Autodesk Fusion 360 part; units mm, degrees
(part 6 of 10)
sketch "草图16 (8)" plane through (0, 0, 19.8) normal (0, 0, 1) x (1, 0, 0) in component "R1_Integrated"
  line L0 (589, 140) -> (725, 140)
  line L1 (725, 140) -> (725, 167)
  line L2 (725, 167) -> (589, 167)
  line L3 (589, 167) -> (589, 140)
  dimension "d2412" = 589
  dimension "d2414" = 136
  dimension "d2415" = 27
  constraint horizontal L0
  constraint vertical L1
  constraint horizontal L2
  constraint vertical L3
  measures "d2412" horizontal distance of origin L0.start
  measures "d2414" horizontal distance of L0.start L0.end
  measures "d2415" vertical distance of L0.end L1.end
extrude "R02 remove projecting spout''" cut sketch "草图16 (8)" along normal blind 20.4 bodies 13 in component "R1_Integrated"
ref_plane "工作平面17" through (593, 0, 0) normal (1, 0, 0) x (0, 1, 0) in component "R1_Integrated"
sketch "草图17 (8)" plane through (593, 0, 0) normal (1, 0, 0) x (0, 0, -1) in component "R1_Integrated"
  line L0 (-24.9649, 136.9) -> (-24.6782, 141)
  line L1 (-24.6782, 141) -> (-41, 141)
  line L2 (-41, 141) -> (-41, 136.9)
  line L3 (-41, 136.9) -> (-24.9649, 136.9)
  dimension "d2420" = 24.9649
  dimension "d2421" = 136.9
  dimension "d2422" = 24.6782
  dimension "d2423" = 141
  dimension "d2424" = 41
  constraint horizontal L1
  constraint vertical L2
  constraint horizontal L3
  measures "d2420" horizontal distance of origin L0.start
  measures "d2421" vertical distance of origin L0.start
  measures "d2422" horizontal distance of origin L0.end
  measures "d2423" vertical distance of origin L0.end
  measures "d2424" horizontal distance of origin L1.end
extrude "R02 full width open front''" cut sketch "草图17 (8)" along normal blind 128 bodies 13 in component "R1_Integrated"
ref_plane "工作平面14" through (0, 0, 36) normal (0, 0, 1) x (1, 0, 0) in component "R1_RemovableGrate"
sketch "草图14 (13)" plane through (0, 0, 36) normal (0, 0, 1) x (1, 0, 0) in component "R1_RemovableGrate"
  line L0 (592.7, 59.7) -> (595.3, 59.7)
  line L1 (595.3, 59.7) -> (595.3, 65.3)
  line L2 (595.3, 65.3) -> (592.7, 65.3)
  line L3 (592.7, 65.3) -> (592.7, 59.7)
  dimension "d2430" = 59.7
  dimension "d2431" = 2.6
  dimension "d2432" = 5.6
  constraint horizontal L0
  constraint vertical L1
  constraint horizontal L2
  constraint vertical L3
  measures "d2430" vertical distance of origin L0.start
  measures "d2431" horizontal distance of L0.start L0.end
  measures "d2432" vertical distance of L0.end L1.end
extrude "R02 side locating notch 0''" cut sketch "草图14 (13)" along normal blind 4 bodies 14 in component "R1_RemovableGrate"
ref_plane "工作平面18" through (0, 0, 20) normal (0, 0, 1) x (1, 0, 0) in component "R1_Integrated"
sketch "草图18 (4)" plane through (0, 0, 20) normal (0, 0, 1) x (1, 0, 0) in component "R1_Integrated"
  line L0 (593, 60) -> (595, 60)
  line L1 (595, 60) -> (595, 65)
  line L2 (595, 65) -> (593, 65)
  line L3 (593, 65) -> (593, 60)
  dimension "d2438" = 60
  dimension "d2439" = 2
  dimension "d2440" = 5
  constraint horizontal L0
  constraint vertical L1
  constraint horizontal L2
  constraint vertical L3
  measures "d2438" vertical distance of origin L0.start
  measures "d2439" horizontal distance of L0.start L0.end
  measures "d2440" vertical distance of L0.end L1.end
extrude "R02 side locating key 0''" add sketch "草图18 (4)" along normal blind 20 bodies 13 in component "R1_Integrated"
ref_plane "工作平面15" through (0, 0, 36) normal (0, 0, 1) x (1, 0, 0) in component "R1_RemovableGrate"
sketch "草图15 (13)" plane through (0, 0, 36) normal (0, 0, 1) x (1, 0, 0) in component "R1_RemovableGrate"
  line L0 (718.7, 59.7) -> (721.3, 59.7)
  line L1 (721.3, 59.7) -> (721.3, 65.3)
  line L2 (721.3, 65.3) -> (718.7, 65.3)
  line L3 (718.7, 65.3) -> (718.7, 59.7)
  dimension "d2445" = 718.7
  dimension "d2446" = 59.7
  dimension "d2447" = 2.6
  dimension "d2448" = 5.6
  constraint horizontal L0
  constraint vertical L1
  constraint horizontal L2
  constraint vertical L3
  measures "d2445" horizontal distance of origin L0.start
  measures "d2446" vertical distance of origin L0.start
  measures "d2447" horizontal distance of L0.start L0.end
  measures "d2448" vertical distance of L0.end L1.end
extrude "R02 side locating notch 1''" cut sketch "草图15 (13)" along normal blind 4 bodies 14 in component "R1_RemovableGrate"
ref_plane "工作平面19" through (0, 0, 20) normal (0, 0, 1) x (1, 0, 0) in component "R1_Integrated"
sketch "草图19 (4)" plane through (0, 0, 20) normal (0, 0, 1) x (1, 0, 0) in component "R1_Integrated"
  line L0 (719, 60) -> (721, 60)
  line L1 (721, 60) -> (721, 65)
  line L2 (721, 65) -> (719, 65)
  line L3 (719, 65) -> (719, 60)
  dimension "d2453" = 719
  dimension "d2454" = 60
  dimension "d2455" = 2
  dimension "d2456" = 5
  constraint horizontal L0
  constraint vertical L1
  constraint horizontal L2
  constraint vertical L3
  measures "d2453" horizontal distance of origin L0.start
  measures "d2454" vertical distance of origin L0.start
  measures "d2455" horizontal distance of L0.start L0.end
  measures "d2456" vertical distance of L0.end L1.end
extrude "R02 side locating key 1''" add sketch "草图19 (4)" along normal blind 20 bodies 13 in component "R1_Integrated"
ref_plane "工作平面16" through (0, 0, 19.8) normal (0, 0, 1) x (1, 0, 0) in component "R2_Integrated"
sketch "草图16 (9)" plane through (0, 0, 19.8) normal (0, 0, 1) x (1, 0, 0) in component "R2_Integrated"
  line L0 (725, 140) -> (861, 140)
  line L1 (861, 140) -> (861, 167)
  line L2 (861, 167) -> (725, 167)
  line L3 (725, 167) -> (725, 140)
  dimension "d2461" = 725
  dimension "d2463" = 136
  dimension "d2464" = 27
  constraint horizontal L0
  constraint vertical L1
  constraint horizontal L2
  constraint vertical L3
  measures "d2461" horizontal distance of origin L0.start
  measures "d2463" horizontal distance of L0.start L0.end
  measures "d2464" vertical distance of L0.end L1.end
extrude "R02 remove projecting spout'''" cut sketch "草图16 (9)" along normal blind 20.4 bodies 19 in component "R2_Integrated"
ref_plane "工作平面17" through (729, 0, 0) normal (1, 0, 0) x (0, 1, 0) in component "R2_Integrated"
sketch "草图17 (9)" plane through (729, 0, 0) normal (1, 0, 0) x (0, 0, -1) in component "R2_Integrated"
  line L0 (-24.9649, 136.9) -> (-24.6782, 141)
  line L1 (-24.6782, 141) -> (-41, 141)
  line L2 (-41, 141) -> (-41, 136.9)
  line L3 (-41, 136.9) -> (-24.9649, 136.9)
  dimension "d2469" = 24.9649
  dimension "d2470" = 136.9
  dimension "d2471" = 24.6782
  dimension "d2472" = 141
  dimension "d2473" = 41
  constraint horizontal L1
  constraint vertical L2
  constraint horizontal L3
  measures "d2469" horizontal distance of origin L0.start
  measures "d2470" vertical distance of origin L0.start
  measures "d2471" horizontal distance of origin L0.end
  measures "d2472" vertical distance of origin L0.end
  measures "d2473" horizontal distance of origin L1.end
extrude "R02 full width open front'''" cut sketch "草图17 (9)" along normal blind 128 bodies 19 in component "R2_Integrated"
ref_plane "工作平面14" through (0, 0, 36) normal (0, 0, 1) x (1, 0, 0) in component "R2_RemovableGrate"
sketch "草图14 (14)" plane through (0, 0, 36) normal (0, 0, 1) x (1, 0, 0) in component "R2_RemovableGrate"
  line L0 (728.7, 59.7) -> (731.3, 59.7)
  line L1 (731.3, 59.7) -> (731.3, 65.3)
  line L2 (731.3, 65.3) -> (728.7, 65.3)
  line L3 (728.7, 65.3) -> (728.7, 59.7)
  dimension "d2478" = 728.7
  dimension "d2479" = 59.7
  dimension "d2480" = 2.6
  dimension "d2481" = 5.6
  constraint horizontal L0
  constraint vertical L1
  constraint horizontal L2
  constraint vertical L3
  measures "d2478" horizontal distance of origin L0.start
  measures "d2479" vertical distance of origin L0.start
  measures "d2480" horizontal distance of L0.start L0.end
  measures "d2481" vertical distance of L0.end L1.end
extrude "R02 side locating notch 0'''" cut sketch "草图14 (14)" along normal blind 4 bodies 20 in component "R2_RemovableGrate"
ref_plane "工作平面18" through (0, 0, 20) normal (0, 0, 1) x (1, 0, 0) in component "R2_Integrated"
sketch "草图18 (5)" plane through (0, 0, 20) normal (0, 0, 1) x (1, 0, 0) in component "R2_Integrated"
  line L0 (729, 60) -> (731, 60)
  line L1 (731, 60) -> (731, 65)
  line L2 (731, 65) -> (729, 65)
  line L3 (729, 65) -> (729, 60)
  dimension "d2486" = 729
  dimension "d2487" = 60
  dimension "d2488" = 2
  dimension "d2489" = 5
  constraint horizontal L0
  constraint vertical L1
  constraint horizontal L2
  constraint vertical L3
  measures "d2486" horizontal distance of origin L0.start
  measures "d2487" vertical distance of origin L0.start
  measures "d2488" horizontal distance of L0.start L0.end
  measures "d2489" vertical distance of L0.end L1.end
extrude "R02 side locating key 0'''" add sketch "草图18 (5)" along normal blind 20 bodies 19 in component "R2_Integrated"
ref_plane "工作平面15" through (0, 0, 36) normal (0, 0, 1) x (1, 0, 0) in component "R2_RemovableGrate"
sketch "草图15 (14)" plane through (0, 0, 36) normal (0, 0, 1) x (1, 0, 0) in component "R2_RemovableGrate"
  line L0 (854.7, 59.7) -> (857.3, 59.7)
  line L1 (857.3, 59.7) -> (857.3, 65.3)
  line L2 (857.3, 65.3) -> (854.7, 65.3)
  line L3 (854.7, 65.3) -> (854.7, 59.7)
  dimension "d2494" = 854.7
  dimension "d2495" = 59.7
  dimension "d2496" = 2.6
  dimension "d2497" = 5.6
  constraint horizontal L0
  constraint vertical L1
  constraint horizontal L2
  constraint vertical L3
  measures "d2494" horizontal distance of origin L0.start
  measures "d2495" vertical distance of origin L0.start
  measures "d2496" horizontal distance of L0.start L0.end
  measures "d2497" vertical distance of L0.end L1.end
extrude "R02 side locating notch 1'''" cut sketch "草图15 (14)" along normal blind 4 bodies 20 in component "R2_RemovableGrate"
ref_plane "工作平面19" through (0, 0, 20) normal (0, 0, 1) x (1, 0, 0) in component "R2_Integrated"
sketch "草图19 (5)" plane through (0, 0, 20) normal (0, 0, 1) x (1, 0, 0) in component "R2_Integrated"
  line L0 (855, 60) -> (857, 60)
  line L1 (857, 60) -> (857, 65)
  line L2 (857, 65) -> (855, 65)
  line L3 (855, 65) -> (855, 60)
  dimension "d2502" = 855
  dimension "d2503" = 60
  dimension "d2504" = 2
  dimension "d2505" = 5
  constraint horizontal L0
  constraint vertical L1
  constraint horizontal L2
  constraint vertical L3
  measures "d2502" horizontal distance of origin L0.start
  measures "d2503" vertical distance of origin L0.start
  measures "d2504" horizontal distance of L0.start L0.end
  measures "d2505" vertical distance of L0.end L1.end
extrude "R02 side locating key 1'''" add sketch "草图19 (5)" along normal blind 20 bodies 19 in component "R2_Integrated"
ref_plane "工作平面16" through (0, 0, 19.8) normal (0, 0, 1) x (1, 0, 0) in component "LS_Integrated"
sketch "草图16 (10)" plane through (0, 0, 19.8) normal (0, 0, 1) x (1, 0, 0) in component "LS_Integrated"
  line L0 (170, 141) -> (197, 141)
  line L1 (197, 141) -> (197, 323)
  line L2 (197, 323) -> (170, 323)
  line L3 (170, 323) -> (170, 141)
  dimension "d2511" = 141
  dimension "d2512" = 27
  dimension "d2513" = 182
  constraint horizontal L0
  constraint vertical L1
  constraint horizontal L2
  constraint vertical L3
  measures "d2511" vertical distance of origin L0.start
  measures "d2512" horizontal distance of L0.start L0.end
  measures "d2513" vertical distance of L0.end L1.end
extrude "R02 remove projecting spout''''" cut sketch "草图16 (10)" along normal blind 20.4 bodies 25 in component "LS_Integrated"
ref_plane "工作平面17" through (0, 319, 0) normal (0, 1, 0) x (0, 0, 1) in component "LS_Integrated"
sketch "草图17 (10)" plane through (0, 319, 0) normal (0, 1, 0) x (1, 0, 0) in component "LS_Integrated"
  line L0 (166.9, -24.9649) -> (171, -24.6782)
  line L1 (171, -24.6782) -> (171, -41)
  line L2 (171, -41) -> (166.9, -41)
  line L3 (166.9, -41) -> (166.9, -24.9649)
  dimension "d2518" = 166.9
  dimension "d2519" = 24.9649
  dimension "d2520" = 171
  dimension "d2521" = 24.6782
  dimension "d2522" = 41
  constraint vertical L1
  constraint horizontal L2
  constraint vertical L3
  measures "d2518" horizontal distance of origin L0.start
  measures "d2519" vertical distance of origin L0.start
  measures "d2520" horizontal distance of origin L0.end
  measures "d2521" vertical distance of origin L0.end
  measures "d2522" vertical distance of origin L1.end
extrude "R02 full width open front''''" cut sketch "草图17 (10)" against normal blind 174 bodies 25 in component "LS_Integrated"
ref_plane "工作平面18" through (0, 0, 36) normal (0, 0, 1) x (1, 0, 0) in component "LS_RemovableGrate"
sketch "草图18 (6)" plane through (0, 0, 36) normal (0, 0, 1) x (1, 0, 0) in component "LS_RemovableGrate"
  line L0 (59.7, 316.7) -> (65.3, 316.7)
  line L1 (65.3, 316.7) -> (65.3, 319.3)
  line L2 (65.3, 319.3) -> (59.7, 319.3)
  line L3 (59.7, 319.3) -> (59.7, 316.7)
  dimension "d2527" = 59.7
  dimension "d2528" = 316.7
  dimension "d2529" = 5.6
  dimension "d2530" = 2.6
  constraint horizontal L0
  constraint vertical L1
  constraint horizontal L2
  constraint vertical L3
  measures "d2527" horizontal distance of origin L0.start
  measures "d2528" vertical distance of origin L0.start
  measures "d2529" horizontal distance of L0.start L0.end
  measures "d2530" vertical distance of L0.end L1.end
extrude "R02 side locating notch 0''''" cut sketch "草图18 (6)" along normal blind 4 bodies 26 in component "LS_RemovableGrate"
ref_plane "工作平面18" through (0, 0, 20) normal (0, 0, 1) x (1, 0, 0) in component "LS_Integrated"
sketch "草图18 (7)" plane through (0, 0, 20) normal (0, 0, 1) x (1, 0, 0) in component "LS_Integrated"
  line L0 (60, 317) -> (65, 317)
  line L1 (65, 317) -> (65, 319)
  line L2 (65, 319) -> (60, 319)
  line L3 (60, 319) -> (60, 317)
  dimension "d2535" = 60
  dimension "d2536" = 317
  dimension "d2537" = 5
  dimension "d2538" = 2
  constraint horizontal L0
  constraint vertical L1
  constraint horizontal L2
  constraint vertical L3
  measures "d2535" horizontal distance of origin L0.start
  measures "d2536" vertical distance of origin L0.start
  measures "d2537" horizontal distance of L0.start L0.end
  measures "d2538" vertical distance of L0.end L1.end
extrude "R02 side locating key 0''''" add sketch "草图18 (7)" along normal blind 20 bodies 25 in component "LS_Integrated"
ref_plane "工作平面19" through (0, 0, 36) normal (0, 0, 1) x (1, 0, 0) in component "LS_RemovableGrate"
sketch "草图19 (6)" plane through (0, 0, 36) normal (0, 0, 1) x (1, 0, 0) in component "LS_RemovableGrate"
  line L0 (59.7, 144.7) -> (65.3, 144.7)
  line L1 (65.3, 144.7) -> (65.3, 147.3)
  line L2 (65.3, 147.3) -> (59.7, 147.3)
  line L3 (59.7, 147.3) -> (59.7, 144.7)
  dimension "d2543" = 59.7
  dimension "d2544" = 144.7
  dimension "d2545" = 5.6
  dimension "d2546" = 2.6
  constraint horizontal L0
  constraint vertical L1
  constraint horizontal L2
  constraint vertical L3
  measures "d2543" horizontal distance of origin L0.start
  measures "d2544" vertical distance of origin L0.start
  measures "d2545" horizontal distance of L0.start L0.end
  measures "d2546" vertical distance of L0.end L1.end
extrude "R02 side locating notch 1''''" cut sketch "草图19 (6)" along normal blind 4 bodies 26 in component "LS_RemovableGrate"
ref_plane "工作平面19" through (0, 0, 20) normal (0, 0, 1) x (1, 0, 0) in component "LS_Integrated"
sketch "草图19 (7)" plane through (0, 0, 20) normal (0, 0, 1) x (1, 0, 0) in component "LS_Integrated"
  line L0 (60, 145) -> (65, 145)
  line L1 (65, 145) -> (65, 147)
  line L2 (65, 147) -> (60, 147)
  line L3 (60, 147) -> (60, 145)
  dimension "d2551" = 60
  dimension "d2552" = 145
  dimension "d2553" = 5
  dimension "d2554" = 2
  constraint horizontal L0
  constraint vertical L1
  constraint horizontal L2
  constraint vertical L3
  measures "d2551" horizontal distance of origin L0.start
  measures "d2552" vertical distance of origin L0.start
  measures "d2553" horizontal distance of L0.start L0.end
  measures "d2554" vertical distance of L0.end L1.end
extrude "R02 side locating key 1''''" add sketch "草图19 (7)" along normal blind 20 bodies 25 in component "LS_Integrated"
ref_plane "工作平面16" through (0, 0, 19.8) normal (0, 0, 1) x (1, 0, 0) in component "RS_Integrated"
sketch "草图16 (11)" plane through (0, 0, 19.8) normal (0, 0, 1) x (1, 0, 0) in component "RS_Integrated"
  line L0 (743, 141) -> (770, 141)
  line L1 (770, 141) -> (770, 323)
  line L2 (770, 323) -> (743, 323)
  line L3 (743, 323) -> (743, 141)
  dimension "d2559" = 743
  dimension "d2560" = 141
  dimension "d2561" = 27
  dimension "d2562" = 182
  constraint horizontal L0
  constraint vertical L1
  constraint horizontal L2
  constraint vertical L3
  measures "d2559" horizontal distance of origin L0.start
  measures "d2560" vertical distance of origin L0.start
  measures "d2561" horizontal distance of L0.start L0.end
  measures "d2562" vertical distance of L0.end L1.end
extrude "R02 remove projecting spout'''''" cut sketch "草图16 (11)" along normal blind 20.4 bodies 31 in component "RS_Integrated"
ref_plane "工作平面17" through (0, 145, 0) normal (0, 1, 0) x (0, 0, 1) in component "RS_Integrated"
sketch "草图17 (11)" plane through (0, 145, 0) normal (0, 1, 0) x (1, 0, 0) in component "RS_Integrated"
  line L0 (773.1, -24.9649) -> (769, -24.6782)
  line L1 (769, -24.6782) -> (769, -41)
  line L2 (769, -41) -> (773.1, -41)
  line L3 (773.1, -41) -> (773.1, -24.9649)
  dimension "d2567" = 773.1
  dimension "d2568" = 24.9649
  dimension "d2569" = 769
  dimension "d2570" = 24.6782
  dimension "d2571" = 41
  constraint vertical L1
  constraint horizontal L2
  constraint vertical L3
  measures "d2567" horizontal distance of origin L0.start
  measures "d2568" vertical distance of origin L0.start
  measures "d2569" horizontal distance of origin L0.end
  measures "d2570" vertical distance of origin L0.end
  measures "d2571" vertical distance of origin L1.end
extrude "R02 full width open front'''''" cut sketch "草图17 (11)" along normal blind 174 bodies 31 in component "RS_Integrated"
ref_plane "工作平面18" through (0, 0, 36) normal (0, 0, 1) x (1, 0, 0) in component "RS_RemovableGrate"
sketch "草图18 (8)" plane through (0, 0, 36) normal (0, 0, 1) x (1, 0, 0) in component "RS_RemovableGrate"
  line L0 (844.7, 144.7) -> (850.3, 144.7)
  line L1 (850.3, 144.7) -> (850.3, 147.3)
  line L2 (850.3, 147.3) -> (844.7, 147.3)
  line L3 (844.7, 147.3) -> (844.7, 144.7)
  dimension "d2576" = 844.7
  dimension "d2578" = 5.6
  dimension "d2579" = 2.6
  constraint horizontal L0
  constraint vertical L1
  constraint horizontal L2
  constraint vertical L3
  measures "d2576" horizontal distance of origin L0.start
  measures "d2578" horizontal distance of L0.start L0.end
  measures "d2579" vertical distance of L0.end L1.end
extrude "R02 side locating notch 0'''''" cut sketch "草图18 (8)" along normal blind 4 bodies 32 in component "RS_RemovableGrate"
ref_plane "工作平面18" through (0, 0, 20) normal (0, 0, 1) x (1, 0, 0) in component "RS_Integrated"
sketch "草图18 (9)" plane through (0, 0, 20) normal (0, 0, 1) x (1, 0, 0) in component "RS_Integrated"
  line L0 (845, 145) -> (850, 145)
  line L1 (850, 145) -> (850, 147)
  line L2 (850, 147) -> (845, 147)
  line L3 (845, 147) -> (845, 145)
  dimension "d2584" = 845
  dimension "d2586" = 5
  dimension "d2587" = 2
  constraint horizontal L0
  constraint vertical L1
  constraint horizontal L2
  constraint vertical L3
  measures "d2584" horizontal distance of origin L0.start
  measures "d2586" horizontal distance of L0.start L0.end
  measures "d2587" vertical distance of L0.end L1.end
extrude "R02 side locating key 0'''''" add sketch "草图18 (9)" along normal blind 20 bodies 31 in component "RS_Integrated"
ref_plane "工作平面19" through (0, 0, 36) normal (0, 0, 1) x (1, 0, 0) in component "RS_RemovableGrate"
sketch "草图19 (8)" plane through (0, 0, 36) normal (0, 0, 1) x (1, 0, 0) in component "RS_RemovableGrate"
  line L0 (844.7, 316.7) -> (850.3, 316.7)
  line L1 (850.3, 316.7) -> (850.3, 319.3)
  line L2 (850.3, 319.3) -> (844.7, 319.3)
  line L3 (844.7, 319.3) -> (844.7, 316.7)
  dimension "d2592" = 844.7
  dimension "d2593" = 316.7
  dimension "d2594" = 5.6
  dimension "d2595" = 2.6
  constraint horizontal L0
  constraint vertical L1
  constraint horizontal L2
  constraint vertical L3
  measures "d2592" horizontal distance of origin L0.start
  measures "d2593" vertical distance of origin L0.start
  measures "d2594" horizontal distance of L0.start L0.end
  measures "d2595" vertical distance of L0.end L1.end
extrude "R02 side locating notch 1'''''" cut sketch "草图19 (8)" along normal blind 4 bodies 32 in component "RS_RemovableGrate"
ref_plane "工作平面19" through (0, 0, 20) normal (0, 0, 1) x (1, 0, 0) in component "RS_Integrated"
sketch "草图19 (9)" plane through (0, 0, 20) normal (0, 0, 1) x (1, 0, 0) in component "RS_Integrated"
  line L0 (845, 317) -> (850, 317)
  line L1 (850, 317) -> (850, 319)
  line L2 (850, 319) -> (845, 319)
  line L3 (845, 319) -> (845, 317)
  dimension "d2600" = 845
  dimension "d2601" = 317
  dimension "d2602" = 5
  dimension "d2603" = 2
  constraint horizontal L0
  constraint vertical L1
  constraint horizontal L2
  constraint vertical L3
  measures "d2600" horizontal distance of origin L0.start
  measures "d2601" vertical distance of origin L0.start
  measures "d2602" horizontal distance of L0.start L0.end
  measures "d2603" vertical distance of L0.end L1.end
extrude "R02 side locating key 1'''''" add sketch "草图19 (9)" along normal blind 20 bodies 31 in component "RS_Integrated"
ref_plane "工作平面16" through (0, 0, 124.8) normal (0, 0, 1) x (1, 0, 0) in component "Tower_Integrated"
sketch "草图16 (12)" plane through (0, 0, 124.8) normal (0, 0, 1) x (1, 0, 0) in component "Tower_Integrated"
  line L0 (49, 140) -> (231, 140)
  line L1 (231, 140) -> (231, 167)
  line L2 (231, 167) -> (49, 167)
  line L3 (49, 167) -> (49, 140)
  dimension "d2608" = 49
  dimension "d2610" = 182
  dimension "d2611" = 27
  constraint horizontal L0
  constraint vertical L1
  constraint horizontal L2
  constraint vertical L3
  measures "d2608" horizontal distance of origin L0.start
  measures "d2610" horizontal distance of L0.start L0.end
  measures "d2611" vertical distance of L0.end L1.end
extrude "R02 remove projecting spout''''''" cut sketch "草图16 (12)" along normal blind 20.4 bodies 37 in component "Tower_Integrated"
ref_plane "工作平面17" through (53, 0, 0) normal (1, 0, 0) x (0, 1, 0) in component "Tower_Integrated"
sketch "草图17 (12)" plane through (53, 0, 0) normal (1, 0, 0) x (0, 0, -1) in component "Tower_Integrated"
  line L0 (-129.9649, 136.9) -> (-129.6782, 141)
  line L1 (-129.6782, 141) -> (-146, 141)
  line L2 (-146, 141) -> (-146, 136.9)
  line L3 (-146, 136.9) -> (-129.9649, 136.9)
  dimension "d2616" = 129.9649
  dimension "d2617" = 136.9
  dimension "d2618" = 129.6782
  dimension "d2619" = 141
  dimension "d2620" = 146
  constraint horizontal L1
  constraint vertical L2
  constraint horizontal L3
  measures "d2616" horizontal distance of origin L0.start
  measures "d2617" vertical distance of origin L0.start
  measures "d2618" horizontal distance of origin L0.end
  measures "d2619" vertical distance of origin L0.end
  measures "d2620" horizontal distance of origin L1.end
extrude "R02 full width open front''''''" cut sketch "草图17 (12)" along normal blind 174 bodies 37 in component "Tower_Integrated"
ref_plane "工作平面18" through (0, 0, 141) normal (0, 0, 1) x (1, 0, 0) in component "UP_RemovableGrate"
sketch "草图18 (10)" plane through (0, 0, 141) normal (0, 0, 1) x (1, 0, 0) in component "UP_RemovableGrate"
  line L0 (52.7, 62.7) -> (55.3, 62.7)
  line L1 (55.3, 62.7) -> (55.3, 68.3)
  line L2 (55.3, 68.3) -> (52.7, 68.3)
  line L3 (52.7, 68.3) -> (52.7, 62.7)
  dimension "d2626" = 62.7
  dimension "d2627" = 2.6
  dimension "d2628" = 5.6
  constraint horizontal L0
  constraint vertical L1
  constraint horizontal L2
  constraint vertical L3
  measures "d2626" vertical distance of origin L0.start
  measures "d2627" horizontal distance of L0.start L0.end
  measures "d2628" vertical distance of L0.end L1.end
extrude "R02 side locating notch 0''''''" cut sketch "草图18 (10)" along normal blind 4 bodies 38 in component "UP_RemovableGrate"
ref_plane "工作平面18" through (0, 0, 125) normal (0, 0, 1) x (1, 0, 0) in component "Tower_Integrated"
sketch "草图18 (11)" plane through (0, 0, 125) normal (0, 0, 1) x (1, 0, 0) in component "Tower_Integrated"
  line L0 (53, 63) -> (55, 63)
  line L1 (55, 63) -> (55, 68)
  line L2 (55, 68) -> (53, 68)
  line L3 (53, 68) -> (53, 63)
  dimension "d2634" = 63
  dimension "d2635" = 2
  dimension "d2636" = 5
  constraint horizontal L0
  constraint vertical L1
  constraint horizontal L2
  constraint vertical L3
  measures "d2634" vertical distance of origin L0.start
  measures "d2635" horizontal distance of L0.start L0.end
  measures "d2636" vertical distance of L0.end L1.end
extrude "R02 side locating key 0''''''" add sketch "草图18 (11)" along normal blind 20 bodies 37 in component "Tower_Integrated"
ref_plane "工作平面19" through (0, 0, 141) normal (0, 0, 1) x (1, 0, 0) in component "UP_RemovableGrate"
sketch "草图19 (10)" plane through (0, 0, 141) normal (0, 0, 1) x (1, 0, 0) in component "UP_RemovableGrate"
  line L0 (224.7, 62.7) -> (227.3, 62.7)
  line L1 (227.3, 62.7) -> (227.3, 68.3)
  line L2 (227.3, 68.3) -> (224.7, 68.3)
  line L3 (224.7, 68.3) -> (224.7, 62.7)
  dimension "d2641" = 224.7
  dimension "d2642" = 62.7
  dimension "d2643" = 2.6
  dimension "d2644" = 5.6
  constraint horizontal L0
  constraint vertical L1
  constraint horizontal L2
  constraint vertical L3
  measures "d2641" horizontal distance of origin L0.start
  measures "d2642" vertical distance of origin L0.start
  measures "d2643" horizontal distance of L0.start L0.end
  measures "d2644" vertical distance of L0.end L1.end
extrude "R02 side locating notch 1''''''" cut sketch "草图19 (10)" along normal blind 4 bodies 38 in component "UP_RemovableGrate"
ref_plane "工作平面19" through (0, 0, 125) normal (0, 0, 1) x (1, 0, 0) in component "Tower_Integrated"
sketch "草图19 (11)" plane through (0, 0, 125) normal (0, 0, 1) x (1, 0, 0) in component "Tower_Integrated"
  line L0 (225, 63) -> (227, 63)
  line L1 (227, 63) -> (227, 68)
  line L2 (227, 68) -> (225, 68)
  line L3 (225, 68) -> (225, 63)
  dimension "d2649" = 225
  dimension "d2650" = 63
  dimension "d2651" = 2
  dimension "d2652" = 5
  constraint horizontal L0
  constraint vertical L1
  constraint horizontal L2
  constraint vertical L3
  measures "d2649" horizontal distance of origin L0.start
  measures "d2650" vertical distance of origin L0.start
  measures "d2651" horizontal distance of L0.start L0.end
  measures "d2652" vertical distance of L0.end L1.end
extrude "R02 side locating key 1''''''" add sketch "草图19 (11)" along normal blind 20 bodies 37 in component "Tower_Integrated"
ref_plane "工作平面20" through (0, 0, 20) normal (0, 0, 1) x (1, 0, 0) in component "L2_Integrated"
sketch "草图20 (2)" plane through (0, 0, 20) normal (0, 0, 1) x (1, 0, 0) in component "L2_Integrated"
  line L0 (238.75, 56.75) -> (247.25, 56.75)
  line L1 (247.25, 56.75) -> (247.25, 65.25)
  line L2 (247.25, 65.25) -> (238.75, 65.25)
  line L3 (238.75, 65.25) -> (238.75, 56.75)
  dimension "d2659" = 238.75
  dimension "d2660" = 56.75
  dimension "d2661" = 8.5
  dimension "d2662" = 8.5
  constraint horizontal L0
  constraint vertical L1
  constraint horizontal L2
  constraint vertical L3
  measures "d2659" horizontal distance of origin L0.start
  measures "d2660" vertical distance of origin L0.start
  measures "d2661" horizontal distance of L0.start L0.end
  measures "d2662" vertical distance of L0.end L1.end
extrude "R03 fill obsolete socket 00" add sketch "草图20 (2)" along normal blind 1.8 bodies 7 in component "L2_Integrated"
ref_plane "工作平面21" through (0, 0, 20) normal (0, 0, 1) x (1, 0, 0) in component "L2_Integrated"
sketch "草图21 (2)" plane through (0, 0, 20) normal (0, 0, 1) x (1, 0, 0) in component "L2_Integrated"
  line L0 (238.75, 118.75) -> (247.25, 118.75)
  line L1 (247.25, 118.75) -> (247.25, 127.25)
  line L2 (247.25, 127.25) -> (238.75, 127.25)
  line L3 (238.75, 127.25) -> (238.75, 118.75)
  dimension "d2667" = 238.75
  dimension "d2668" = 118.75
  dimension "d2669" = 8.5
  dimension "d2670" = 8.5
  constraint horizontal L0
  constraint vertical L1
  constraint horizontal L2
  constraint vertical L3
  measures "d2667" horizontal distance of origin L0.start
  measures "d2668" vertical distance of origin L0.start
  measures "d2669" horizontal distance of L0.start L0.end
  measures "d2670" vertical distance of L0.end L1.end
extrude "R03 fill obsolete socket 01" add sketch "草图21 (2)" along normal blind 1.8 bodies 7 in component "L2_Integrated"
ref_plane "工作平面22" through (0, 0, 20) normal (0, 0, 1) x (1, 0, 0) in component "L2_Integrated"
sketch "草图22" plane through (0, 0, 20) normal (0, 0, 1) x (1, 0, 0) in component "L2_Integrated"
  line L0 (414.75, 56.75) -> (423.25, 56.75)
  line L1 (423.25, 56.75) -> (423.25, 65.25)
  line L2 (423.25, 65.25) -> (414.75, 65.25)
  line L3 (414.75, 65.25) -> (414.75, 56.75)
  dimension "d2675" = 414.75
  dimension "d2676" = 56.75
  dimension "d2677" = 8.5
  dimension "d2678" = 8.5
  constraint horizontal L0
  constraint vertical L1
  constraint horizontal L2
  constraint vertical L3
  measures "d2675" horizontal distance of origin L0.start
  measures "d2676" vertical distance of origin L0.start
  measures "d2677" horizontal distance of L0.start L0.end
  measures "d2678" vertical distance of L0.end L1.end
extrude "R03 fill obsolete socket 10" add sketch "草图22" along normal blind 1.8 bodies 7 in component "L2_Integrated"
ref_plane "工作平面23" through (0, 0, 20) normal (0, 0, 1) x (1, 0, 0) in component "L2_Integrated"
sketch "草图23" plane through (0, 0, 20) normal (0, 0, 1) x (1, 0, 0) in component "L2_Integrated"
  line L0 (414.75, 118.75) -> (423.25, 118.75)
  line L1 (423.25, 118.75) -> (423.25, 127.25)
  line L2 (423.25, 127.25) -> (414.75, 127.25)
  line L3 (414.75, 127.25) -> (414.75, 118.75)
  dimension "d2683" = 414.75
  dimension "d2684" = 118.75
  dimension "d2685" = 8.5
  dimension "d2686" = 8.5
  constraint horizontal L0
  constraint vertical L1
  constraint horizontal L2
  constraint vertical L3
  measures "d2683" horizontal distance of origin L0.start
  measures "d2684" vertical distance of origin L0.start
  measures "d2685" horizontal distance of L0.start L0.end
  measures "d2686" vertical distance of L0.end L1.end
extrude "R03 fill obsolete socket 11" add sketch "草图23" along normal blind 1.8 bodies 7 in component "L2_Integrated"
ref_plane "工作平面24" through (0, 0, 0) normal (0, 0, 1) x (1, 0, 0) in component "L2_Integrated"
sketch "草图24" plane through (0, 0, 0) normal (0, 0, 1) x (1, 0, 0) in component "L2_Integrated"
  line L0 (235, 50) -> (243, 50)
  line L1 (243, 50) -> (243, 131)
  line L2 (243, 131) -> (235, 131)
  line L3 (235, 131) -> (235, 50)
  dimension "d2691" = 235
  dimension "d2692" = 50
  dimension "d2693" = 8
  dimension "d2694" = 81
  constraint horizontal L0
  constraint vertical L1
  constraint horizontal L2
  constraint vertical L3
  measures "d2691" horizontal distance of origin L0.start
  measures "d2692" vertical distance of origin L0.start
  measures "d2693" horizontal distance of L0.start L0.end
  measures "d2694" vertical distance of L0.end L1.end
extrude "R03 integral runner 0" add sketch "草图24" along normal blind 20 bodies 7 in component "L2_Integrated"
ref_plane "工作平面25" through (0, 0, 0) normal (0, 0, 1) x (1, 0, 0) in component "L2_Integrated"
sketch "草图25" plane through (0, 0, 0) normal (0, 0, 1) x (1, 0, 0) in component "L2_Integrated"
  line L0 (419, 50) -> (427, 50)
  line L1 (427, 50) -> (427, 131)
  line L2 (427, 131) -> (419, 131)
  line L3 (419, 131) -> (419, 50)
  dimension "d2699" = 419
  dimension "d2700" = 50
  dimension "d2701" = 8
  dimension "d2702" = 81
  constraint horizontal L0
  constraint vertical L1
  constraint horizontal L2
  constraint vertical L3
  measures "d2699" horizontal distance of origin L0.start
  measures "d2700" vertical distance of origin L0.start
  measures "d2701" horizontal distance of L0.start L0.end
  measures "d2702" vertical distance of L0.end L1.end
extrude "R03 integral runner 1" add sketch "草图25" along normal blind 20 bodies 7 in component "L2_Integrated"
chamfer "R03 touch edge chamfer" distance 0.4 angle 45 5 edges at (427, 102.5, 40) (235, 102.5, 40) (331, 53, 40) (232, 95, 40) (430, 95, 40) on bodies 7 in component "L2_Integrated"
ref_plane "工作平面20" through (0, 0, 20) normal (0, 0, 1) x (1, 0, 0) in component "L1_DrainPan"
sketch "草图20 (3)" plane through (0, 0, 20) normal (0, 0, 1) x (1, 0, 0) in component "L1_DrainPan"
  line L0 (66.75, 56.75) -> (75.25, 56.75)
  line L1 (75.25, 56.75) -> (75.25, 65.25)
  line L2 (75.25, 65.25) -> (66.75, 65.25)
  line L3 (66.75, 65.25) -> (66.75, 56.75)
  dimension "d2708" = 66.75
  dimension "d2709" = 56.75
  dimension "d2710" = 8.5
  dimension "d2711" = 8.5
  constraint horizontal L0
  constraint vertical L1
  constraint horizontal L2
  constraint vertical L3
  measures "d2708" horizontal distance of origin L0.start
  measures "d2709" vertical distance of origin L0.start
  measures "d2710" horizontal distance of L0.start L0.end
  measures "d2711" vertical distance of L0.end L1.end
extrude "R03 fill obsolete socket 00'" add sketch "草图20 (3)" along normal blind 1.8 bodies 1 in component "L1_DrainPan"
ref_plane "工作平面21" through (0, 0, 20) normal (0, 0, 1) x (1, 0, 0) in component "L1_DrainPan"
sketch "草图21 (3)" plane through (0, 0, 20) normal (0, 0, 1) x (1, 0, 0) in component "L1_DrainPan"
  line L0 (66.75, 118.75) -> (75.25, 118.75)
  line L1 (75.25, 118.75) -> (75.25, 127.25)
  line L2 (75.25, 127.25) -> (66.75, 127.25)
  line L3 (66.75, 127.25) -> (66.75, 118.75)
  dimension "d2716" = 66.75
  dimension "d2717" = 118.75
  dimension "d2718" = 8.5
  dimension "d2719" = 8.5
  constraint horizontal L0
  constraint vertical L1
  constraint horizontal L2
  constraint vertical L3
  measures "d2716" horizontal distance of origin L0.start
  measures "d2717" vertical distance of origin L0.start
  measures "d2718" horizontal distance of L0.start L0.end
  measures "d2719" vertical distance of L0.end L1.end
extrude "R03 fill obsolete socket 01'" add sketch "草图21 (3)" along normal blind 1.8 bodies 1 in component "L1_DrainPan"
ref_plane "工作平面22" through (0, 0, 20) normal (0, 0, 1) x (1, 0, 0) in component "L1_DrainPan"
sketch "草图22 (2)" plane through (0, 0, 20) normal (0, 0, 1) x (1, 0, 0) in component "L1_DrainPan"
  line L0 (204.75, 56.75) -> (213.25, 56.75)
  line L1 (213.25, 56.75) -> (213.25, 65.25)
  line L2 (213.25, 65.25) -> (204.75, 65.25)
  line L3 (204.75, 65.25) -> (204.75, 56.75)
  dimension "d2724" = 204.75
  dimension "d2725" = 56.75
  dimension "d2726" = 8.5
  dimension "d2727" = 8.5
  constraint horizontal L0
  constraint vertical L1
  constraint horizontal L2
  constraint vertical L3
  measures "d2724" horizontal distance of origin L0.start
  measures "d2725" vertical distance of origin L0.start
  measures "d2726" horizontal distance of L0.start L0.end
  measures "d2727" vertical distance of L0.end L1.end
extrude "R03 fill obsolete socket 10'" add sketch "草图22 (2)" along normal blind 1.8 bodies 1 in component "L1_DrainPan"
ref_plane "工作平面23" through (0, 0, 20) normal (0, 0, 1) x (1, 0, 0) in component "L1_DrainPan"
sketch "草图23 (2)" plane through (0, 0, 20) normal (0, 0, 1) x (1, 0, 0) in component "L1_DrainPan"
  line L0 (204.75, 118.75) -> (213.25, 118.75)
  line L1 (213.25, 118.75) -> (213.25, 127.25)
  line L2 (213.25, 127.25) -> (204.75, 127.25)
  line L3 (204.75, 127.25) -> (204.75, 118.75)
  dimension "d2732" = 204.75
  dimension "d2733" = 118.75
  dimension "d2734" = 8.5
  dimension "d2735" = 8.5
  constraint horizontal L0
  constraint vertical L1
  constraint horizontal L2
  constraint vertical L3
  measures "d2732" horizontal distance of origin L0.start
  measures "d2733" vertical distance of origin L0.start
  measures "d2734" horizontal distance of L0.start L0.end
  measures "d2735" vertical distance of L0.end L1.end
extrude "R03 fill obsolete socket 11'" add sketch "草图23 (2)" along normal blind 1.8 bodies 1 in component "L1_DrainPan"
ref_plane "工作平面20" through (0, 0, 0) normal (0, 0, 1) x (1, 0, 0) in component "Tower_Integrated"
sketch "草图20 (4)" plane through (0, 0, 0) normal (0, 0, 1) x (1, 0, 0) in component "Tower_Integrated"
  line L0 (50, 50) -> (58, 50)
  line L1 (58, 50) -> (58, 140)
  line L2 (58, 140) -> (50, 140)
  line L3 (50, 140) -> (50, 50)
  dimension "d2740" = 50
  dimension "d2741" = 50
  dimension "d2742" = 8
  dimension "d2743" = 90
  constraint horizontal L0
  constraint vertical L1
  constraint horizontal L2
  constraint vertical L3
  measures "d2740" horizontal distance of origin L0.start
  measures "d2741" vertical distance of origin L0.start
  measures "d2742" horizontal distance of L0.start L0.end
  measures "d2743" vertical distance of L0.end L1.end
extrude "R03 integral side panel 0" add sketch "草图20 (4)" along normal blind 127 bodies 37 in component "Tower_Integrated"
ref_plane "工作平面21" through (0, 0, 0) normal (0, 0, 1) x (1, 0, 0) in component "Tower_Integrated"
sketch "草图21 (4)" plane through (0, 0, 0) normal (0, 0, 1) x (1, 0, 0) in component "Tower_Integrated"
  line L0 (222, 50) -> (230, 50)
  line L1 (230, 50) -> (230, 140)
  line L2 (230, 140) -> (222, 140)
  line L3 (222, 140) -> (222, 50)
  dimension "d2748" = 222
  dimension "d2749" = 50
  dimension "d2750" = 8
  dimension "d2751" = 90
  constraint horizontal L0
  constraint vertical L1
  constraint horizontal L2
  constraint vertical L3
  measures "d2748" horizontal distance of origin L0.start
  measures "d2749" vertical distance of origin L0.start
  measures "d2750" horizontal distance of L0.start L0.end
  measures "d2751" vertical distance of L0.end L1.end
extrude "R03 integral side panel 1" add sketch "草图21 (4)" along normal blind 127 bodies 37 in component "Tower_Integrated"
ref_plane "工作平面22" through (0, 0, 20) normal (0, 0, 1) x (1, 0, 0) in component "Tower_Integrated"
sketch "草图22 (3)" plane through (0, 0, 20) normal (0, 0, 1) x (1, 0, 0) in component "Tower_Integrated"
  line L0 (58, 50) -> (60, 50)
  line L1 (60, 50) -> (60, 140)
  line L2 (60, 140) -> (58, 140)
  line L3 (58, 140) -> (58, 50)
  dimension "d2756" = 58
  dimension "d2757" = 50
  dimension "d2758" = 2
  dimension "d2759" = 90
  constraint horizontal L0
  constraint vertical L1
  constraint horizontal L2
  constraint vertical L3
  measures "d2756" horizontal distance of origin L0.start
  measures "d2757" vertical distance of origin L0.start
  measures "d2758" horizontal distance of L0.start L0.end
  measures "d2759" vertical distance of L0.end L1.end
extrude "R03 lower tray connection 0" add sketch "草图22 (3)" along normal blind 20 bodies 37 in component "Tower_Integrated"
ref_plane "工作平面23" through (0, 0, 20) normal (0, 0, 1) x (1, 0, 0) in component "Tower_Integrated"
sketch "草图23 (3)" plane through (0, 0, 20) normal (0, 0, 1) x (1, 0, 0) in component "Tower_Integrated"
  line L0 (220, 50) -> (222, 50)
  line L1 (222, 50) -> (222, 140)
  line L2 (222, 140) -> (220, 140)
  line L3 (220, 140) -> (220, 50)
  dimension "d2764" = 220
  dimension "d2765" = 50
  dimension "d2766" = 2
  dimension "d2767" = 90
  constraint horizontal L0
  constraint vertical L1
  constraint horizontal L2
  constraint vertical L3
  measures "d2764" horizontal distance of origin L0.start
  measures "d2765" vertical distance of origin L0.start
  measures "d2766" horizontal distance of L0.start L0.end
  measures "d2767" vertical distance of L0.end L1.end
extrude "R03 lower tray connection 1" add sketch "草图23 (3)" along normal blind 20 bodies 37 in component "Tower_Integrated"
combine "R03 integrated upper and lower tower" operation add target body 37 tool bodies 1 in component "Tower_Integrated"
chamfer "R03 touch edge chamfer'" distance 0.4 angle 45 5 edges at (227, 104, 145) (53, 104, 145) (140, 53, 145) (50, 95, 145) (230, 95, 145) on bodies 37 in component "Tower_Integrated"
ref_plane "工作平面20" through (0, 0, 20) normal (0, 0, 1) x (1, 0, 0) in component "R1_Integrated"
sketch "草图20 (5)" plane through (0, 0, 20) normal (0, 0, 1) x (1, 0, 0) in component "R1_Integrated"
  line L0 (596.75, 56.75) -> (605.25, 56.75)
  line L1 (605.25, 56.75) -> (605.25, 65.25)
  line L2 (605.25, 65.25) -> (596.75, 65.25)
  line L3 (596.75, 65.25) -> (596.75, 56.75)
  dimension "d2773" = 596.75
  dimension "d2774" = 56.75
  dimension "d2775" = 8.5
  dimension "d2776" = 8.5
  constraint horizontal L0
  constraint vertical L1
  constraint horizontal L2
  constraint vertical L3
  measures "d2773" horizontal distance of origin L0.start
  measures "d2774" vertical distance of origin L0.start
  measures "d2775" horizontal distance of L0.start L0.end
  measures "d2776" vertical distance of L0.end L1.end
extrude "R03 fill obsolete socket 00''" add sketch "草图20 (5)" along normal blind 1.8 bodies 13 in component "R1_Integrated"
ref_plane "工作平面21" through (0, 0, 20) normal (0, 0, 1) x (1, 0, 0) in component "R1_Integrated"
sketch "草图21 (5)" plane through (0, 0, 20) normal (0, 0, 1) x (1, 0, 0) in component "R1_Integrated"
  line L0 (596.75, 118.75) -> (605.25, 118.75)
  line L1 (605.25, 118.75) -> (605.25, 127.25)
  line L2 (605.25, 127.25) -> (596.75, 127.25)
  line L3 (596.75, 127.25) -> (596.75, 118.75)
  dimension "d2781" = 596.75
  dimension "d2782" = 118.75
  dimension "d2783" = 8.5
  dimension "d2784" = 8.5
  constraint horizontal L0
  constraint vertical L1
  constraint horizontal L2
  constraint vertical L3
  measures "d2781" horizontal distance of origin L0.start
  measures "d2782" vertical distance of origin L0.start
  measures "d2783" horizontal distance of L0.start L0.end
  measures "d2784" vertical distance of L0.end L1.end
extrude "R03 fill obsolete socket 01''" add sketch "草图21 (5)" along normal blind 1.8 bodies 13 in component "R1_Integrated"
ref_plane "工作平面22" through (0, 0, 20) normal (0, 0, 1) x (1, 0, 0) in component "R1_Integrated"
sketch "草图22 (4)" plane through (0, 0, 20) normal (0, 0, 1) x (1, 0, 0) in component "R1_Integrated"
  line L0 (708.75, 56.75) -> (717.25, 56.75)
  line L1 (717.25, 56.75) -> (717.25, 65.25)
  line L2 (717.25, 65.25) -> (708.75, 65.25)
  line L3 (708.75, 65.25) -> (708.75, 56.75)
  dimension "d2789" = 708.75
  dimension "d2790" = 56.75
  dimension "d2791" = 8.5
  dimension "d2792" = 8.5
  constraint horizontal L0
  constraint vertical L1
  constraint horizontal L2
  constraint vertical L3
  measures "d2789" horizontal distance of origin L0.start
  measures "d2790" vertical distance of origin L0.start
  measures "d2791" horizontal distance of L0.start L0.end
  measures "d2792" vertical distance of L0.end L1.end
extrude "R03 fill obsolete socket 10''" add sketch "草图22 (4)" along normal blind 1.8 bodies 13 in component "R1_Integrated"
ref_plane "工作平面23" through (0, 0, 20) normal (0, 0, 1) x (1, 0, 0) in component "R1_Integrated"
sketch "草图23 (4)" plane through (0, 0, 20) normal (0, 0, 1) x (1, 0, 0) in component "R1_Integrated"
  line L0 (708.75, 118.75) -> (717.25, 118.75)
  line L1 (717.25, 118.75) -> (717.25, 127.25)
  line L2 (717.25, 127.25) -> (708.75, 127.25)
  line L3 (708.75, 127.25) -> (708.75, 118.75)
  dimension "d2797" = 708.75
  dimension "d2798" = 118.75
  dimension "d2799" = 8.5
  dimension "d2800" = 8.5
  constraint horizontal L0
  constraint vertical L1
  constraint horizontal L2
  constraint vertical L3
  measures "d2797" horizontal distance of origin L0.start
  measures "d2798" vertical distance of origin L0.start
  measures "d2799" horizontal distance of L0.start L0.end
  measures "d764" distance of L0.end L1.end
extrude "R03 fill obsolete socket 11''" add sketch "草图23 (4)" along normal blind 1.8 bodies 13 in component "R1_Integrated"
ref_plane "工作平面24" through (0, 0, 0) normal (0, 0, 1) x (1, 0, 0) in component "R1_Integrated"
sketch "草图24 (2)" plane through (0, 0, 0) normal (0, 0, 1) x (1, 0, 0) in component "R1_Integrated"
  line L0 (593, 50) -> (601, 50)
  line L1 (601, 50) -> (601, 131)
  line L2 (601, 131) -> (593, 131)
  line L3 (593, 131) -> (593, 50)
  dimension "d2805" = 593
  dimension "d2806" = 50
  dimension "d2807" = 8
  dimension "d2808" = 81
  constraint horizontal L0
  constraint vertical L1
  constraint horizontal L2
  constraint vertical L3
  measures "d2805" horizontal distance of origin L0.start
  measures "d2806" vertical distance of origin L0.start
  measures "d2807" horizontal distance of L0.start L0.end
  measures "d2808" vertical distance of L0.end L1.end
extrude "R03 integral runner 0'" add sketch "草图24 (2)" along normal blind 20 bodies 13 in component "R1_Integrated"
ref_plane "工作平面25" through (0, 0, 0) normal (0, 0, 1) x (1, 0, 0) in component "R1_Integrated"
sketch "草图25 (2)" plane through (0, 0, 0) normal (0, 0, 1) x (1, 0, 0) in component "R1_Integrated"
  line L0 (713, 50) -> (721, 50)
  line L1 (721, 50) -> (721, 131)
  line L2 (721, 131) -> (713, 131)
  line L3 (713, 131) -> (713, 50)
  dimension "d2813" = 713
  dimension "d2814" = 50
  dimension "d2815" = 8
  dimension "d2816" = 81
  constraint horizontal L0
  constraint vertical L1
  constraint horizontal L2
  constraint vertical L3
  measures "d2813" horizontal distance of origin L0.start
  measures "d2814" vertical distance of origin L0.start
  measures "d2815" horizontal distance of L0.start L0.end
  measures "d2816" vertical distance of L0.end L1.end
extrude "R03 integral runner 1'" add sketch "草图25 (2)" along normal blind 20 bodies 13 in component "R1_Integrated"
chamfer "R03 touch edge chamfer''" distance 0.4 angle 45 5 edges at (721, 102.5, 40) (593, 102.5, 40) (657, 53, 40) (590, 95, 40) (724, 95, 40) on bodies 13 in component "R1_Integrated"
ref_plane "工作平面20" through (0, 0, 20) normal (0, 0, 1) x (1, 0, 0) in component "R2_Integrated"
sketch "草图20 (6)" plane through (0, 0, 20) normal (0, 0, 1) x (1, 0, 0) in component "R2_Integrated"
  line L0 (732.75, 56.75) -> (741.25, 56.75)
  line L1 (741.25, 56.75) -> (741.25, 65.25)
  line L2 (741.25, 65.25) -> (732.75, 65.25)
  line L3 (732.75, 65.25) -> (732.75, 56.75)
  dimension "d2822" = 732.75
  dimension "d2823" = 56.75
  dimension "d2824" = 8.5
  dimension "d2825" = 8.5
  constraint horizontal L0
  constraint vertical L1
  constraint horizontal L2
  constraint vertical L3
  measures "d2822" horizontal distance of origin L0.start
  measures "d2823" vertical distance of origin L0.start
  measures "d2824" horizontal distance of L0.start L0.end
  measures "d2825" vertical distance of L0.end L1.end
extrude "R03 fill obsolete socket 00'''" add sketch "草图20 (6)" along normal blind 1.8 bodies 19 in component "R2_Integrated"
ref_plane "工作平面21" through (0, 0, 20) normal (0, 0, 1) x (1, 0, 0) in component "R2_Integrated"
sketch "草图21 (6)" plane through (0, 0, 20) normal (0, 0, 1) x (1, 0, 0) in component "R2_Integrated"
  line L0 (732.75, 118.75) -> (741.25, 118.75)
  line L1 (741.25, 118.75) -> (741.25, 127.25)
  line L2 (741.25, 127.25) -> (732.75, 127.25)
  line L3 (732.75, 127.25) -> (732.75, 118.75)
  dimension "d2830" = 732.75
  dimension "d2831" = 118.75
  dimension "d2832" = 8.5
  dimension "d2833" = 8.5
  constraint horizontal L0
  constraint vertical L1
  constraint horizontal L2
  constraint vertical L3
  measures "d2830" horizontal distance of origin L0.start
  measures "d2831" vertical distance of origin L0.start
  measures "d2832" horizontal distance of L0.start L0.end
  measures "d2833" vertical distance of L0.end L1.end
extrude "R03 fill obsolete socket 01'''" add sketch "草图21 (6)" along normal blind 1.8 bodies 19 in component "R2_Integrated"
ref_plane "工作平面22" through (0, 0, 20) normal (0, 0, 1) x (1, 0, 0) in component "R2_Integrated"
sketch "草图22 (5)" plane through (0, 0, 20) normal (0, 0, 1) x (1, 0, 0) in component "R2_Integrated"
  line L0 (844.75, 56.75) -> (853.25, 56.75)
  line L1 (853.25, 56.75) -> (853.25, 65.25)
  line L2 (853.25, 65.25) -> (844.75, 65.25)
  line L3 (844.75, 65.25) -> (844.75, 56.75)
  dimension "d2838" = 844.75
  dimension "d2839" = 56.75
  dimension "d2840" = 8.5
  dimension "d2841" = 8.5
  constraint horizontal L0
  constraint vertical L1
  constraint horizontal L2
  constraint vertical L3
  measures "d2838" horizontal distance of origin L0.start
  measures "d2839" vertical distance of origin L0.start
  measures "d2840" horizontal distance of L0.start L0.end
  measures "d2841" vertical distance of L0.end L1.end
extrude "R03 fill obsolete socket 10'''" add sketch "草图22 (5)" along normal blind 1.8 bodies 19 in component "R2_Integrated"
ref_plane "工作平面23" through (0, 0, 20) normal (0, 0, 1) x (1, 0, 0) in component "R2_Integrated"
sketch "草图23 (5)" plane through (0, 0, 20) normal (0, 0, 1) x (1, 0, 0) in component "R2_Integrated"
  line L0 (844.75, 118.75) -> (853.25, 118.75)
  line L1 (853.25, 118.75) -> (853.25, 127.25)
  line L2 (853.25, 127.25) -> (844.75, 127.25)
  line L3 (844.75, 127.25) -> (844.75, 118.75)
  dimension "d2846" = 844.75
  dimension "d2847" = 118.75
  dimension "d2848" = 8.5
  dimension "d2849" = 8.5
  constraint horizontal L0
  constraint vertical L1
  constraint horizontal L2
  constraint vertical L3
  measures "d2846" horizontal distance of origin L0.start
  measures "d2847" vertical distance of origin L0.start
  measures "d2848" horizontal distance of L0.start L0.end
  measures "d2849" vertical distance of L0.end L1.end
extrude "R03 fill obsolete socket 11'''" add sketch "草图23 (5)" along normal blind 1.8 bodies 19 in component "R2_Integrated"
ref_plane "工作平面24" through (0, 0, 0) normal (0, 0, 1) x (1, 0, 0) in component "R2_Integrated"